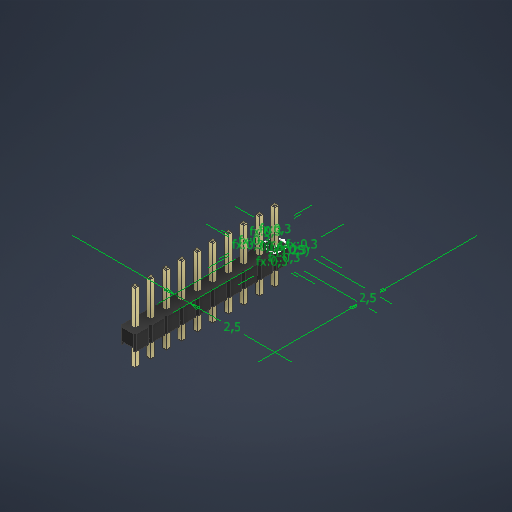
# Autodesk Inventor part: BarraPinosv2
Saved by Autodesk Inventor 2027 (Build 310192060, 192F)
## iProperties
Created: 2026-06-25
Part Number: BarraPinosv2
Material: Genérico
Document SubType Name: Modeling
Designer: EspacoMaker
Density: 1 g/cm^3
Appearance: Padrão
Author: EspacoMaker
Autodesk Inventor part; units mm, degrees
ref_plane "YZ Plane" through (0, 0, 0) normal (1, 0, 0) x (0, 1, 0)
ref_plane "XZ Plane" through (0, 0, 0) normal (0, 1, 0) x (-1, 0, 0)
ref_plane "XY Plane" through (0, 0, 0) normal (0, 0, 1) x (1, 0, 0)
sketch "Esboço1" plane through (0, 0, 0) normal (0, 1, 0) x (-1, 0, 0)
  line L0 (0.95, -1.25) -> (-0.95, -1.25)
  line L1 (-1.25, -0.95) -> (-1.25, 0.95)
  line L2 (-0.95, 1.25) -> (0.95, 1.25)
  line L3 (1.25, 0.95) -> (1.25, -0.95)
  line L4 (1.25, -1.25) -> (-1.25, 1.25) construction
  line L5 (-1.25, -1.25) -> (1.25, 1.25) construction
  line L6 (-1.25, -0.95) -> (-0.95, -1.25)
  line L7 (1.25, -0.95) -> (0.95, -1.25)
  line L8 (0.95, 1.25) -> (1.25, 0.95)
  line L9 (-1.25, 0.95) -> (-0.95, 1.25)
  line L10 (0.32, -0.32) -> (-0.32, -0.32)
  line L11 (-0.32, -0.32) -> (-0.32, 0.32)
  line L12 (-0.32, 0.32) -> (0.32, 0.32)
  line L13 (0.32, 0.32) -> (0.32, -0.32)
  line L14 (0.32, -0.32) -> (-0.32, 0.32) construction
  line L15 (-0.32, -0.32) -> (0.32, 0.32) construction
  line L16 (0.275, -0.275) -> (-0.275, 0.275) construction
  line L17 (-0.275, -0.275) -> (0.275, 0.275) construction
  point P0 (0, 0)
  point P1 (0, -1.25)
  dimension "d0" = 2.5
  dimension "d1" = 2.5
  dimension "d2" = 0.3
  dimension "d3" = 0.3
  dimension "d4" = 0.3
  dimension "d5" = 0.3
  dimension "d6" = 0.3
  dimension "d7" = 0.3
  dimension "d8" = 0.3
  dimension "d9" = 0.3
  dimension "d10" = 0.64
  dimension "d11" = 0.64
  dimension "d36" = 1.25
  constraints: 36 end point, 9 point on line, 7 midpoint, 4 parallel, 2 horizontal, 2 perpendicular
  measures "d0" distance of L4.end L5.end
  measures "d1" distance of L5.start L4.end
  measures "d2" distance of L1.start L5.start
  measures "d3" distance of L0.end L5.start
  measures "d4" distance of L3.end L4.start
  measures "d5" distance of L0.start L4.start
  measures "d6" distance of L2.end L5.end
  measures "d7" distance of L3.start L5.end
  measures "d8" distance of L1.end L4.end
  measures "d9" distance of L2.start L4.end
  measures "d10" distance of L11.end L12.end
  measures "d11" distance of L10.end L11.end
  measures "d36" distance of point (0, -1.25) point (0, 0)
extrude "Extrusão1" add sketch "Esboço1" against normal blind 2.5 contours L0 L6 L1 L9 L2 L8 L3 L7 | L10 L11 L12 L13
sketch "Esboço3" plane through (-0.95, 0, 1.25) normal (0, 0, 1) x (1, 0, 0)
  line L0 (0, -2.5) -> (-0.3, -2.5) projected
  line L1 (1.9, 0) -> (1.9, -2.5) projected
  line L2 (0, -2.5) -> (1.9, -2.5)
  line L3 (1.9, -2.5) -> (1.9, -2)
  line L4 (1.9, -2) -> (0, -2)
  line L5 (0, -2) -> (0, -2.5)
  point P0 (0.95, 0)
  dimension "d25" = 0.5
  constraints: 8 end point, 2 parallel, 1 horizontal, 1 perpendicular, 1 point on line
  measures "d25" distance of L3.end L2.end
extrude "Extrusão3" cut sketch "Esboço3" against normal blind 11.55
extrude "Extrusão4" add sketch "Esboço1" along normal mid plane 11.55 contours L10 L11 L12 L13
chamfer "Chanfro3" distance 0.09 angle 60 4 edges at (-0.32, 5.775, 0) (0, 5.775, -0.32) (0.32, 5.775, 0) (0, 5.775, 0.32) measured on face at (0.1067, 5.775, 0.1067)
chamfer "Chanfro4" distance 0.09 angle 60 4 edges at (0.32, -5.775, 0) (0, -5.775, -0.32) (-0.32, -5.775, 0) (0, -5.775, 0.32) measured on face at (0.1067, -5.775, 0.1067)
sketch "Esboço4" plane through (-0.95, 0, 1.25) normal (0, 0, 1) x (1, 0, 0)
  line L0 (1.9, 0) -> (0, 0) projected
  line L1 (0, 0) -> (1.9, 0)
  line L2 (1.9, 0) -> (1.9, -2)
  line L3 (1.9, -2) -> (0, -2)
  line L4 (0, -2) -> (0, 0)
  point P0 (0.95, 0)
  constraints: 8 end point, 2 parallel, 1 horizontal, 1 perpendicular
extrude "Extrusão5" add sketch "Esboço4" along normal blind 0.04
pattern_linear "Rectangular Pattern2" count 10 spacing 2.54 along (0, 0, 1) of "Extrusão1", "Extrusão3", "Extrusão4", "Chanfro3", "Chanfro4", "Extrusão5"
equation "\"d3\" = d2"
equation "\"d4\" = d2"
equation "\"d5\" = d4"
equation "\"d6\" = d2"
equation "\"d7\" = d6"
equation "\"d8\" = d2"
equation "\"d9\" = d8"
